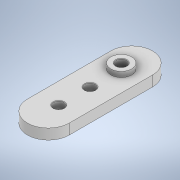
# Autodesk Inventor part: Board
Saved by Autodesk Inventor 2022 (Build 260153000, 153)
## iProperties
Created: 2021-09-18
Part Number: Board
Material: Generic
Document SubType Name: Modeling
Designer: marcu
Density: 1 g/cm^3
Appearance: Default
Author: marcu
Autodesk Inventor part; units mm, degrees
ref_plane "YZ Plane" through (0, 0, 0) normal (1, 0, 0) x (0, 1, 0)
ref_plane "XZ Plane" through (0, 0, 0) normal (0, 1, 0) x (-1, 0, 0)
ref_plane "XY Plane" through (0, 0, 0) normal (0, 0, 1) x (1, 0, 0)
sketch "Sketch1" plane through (0, 0, 0) normal (0, 1, 0) x (-1, 0, 0)
  line L0 (0, 0) -> (25.4, 0)
  line L1 (25.4, 0) -> (25.4, -76.2)
  line L2 (25.4, -76.2) -> (0, -76.2)
  line L3 (0, -76.2) -> (0, 0)
  dimension "d0" = 25.4
  dimension "d1" = 76.2
  constraints: 8 end point, 2 parallel, 1 horizontal, 1 perpendicular
  measures "d0" distance of L1.end L2.end
  measures "d1" distance of L0.end L1.end
extrude "Extrusion1" add sketch "Sketch1" along normal blind 3.175
sketch "Sketch2" plane through (0, 3.175, 0) normal (0, 1, 0) x (1, 0, 0)
  line L0 (-25.4, 76.2) -> (-25.4, 0) projected
  line L1 (0, 76.2) -> (-25.4, 76.2) projected
  line L2 (-25.4, 0) -> (0, 76.2)
  line L3 (0, 76.2) -> (-25.4, 76.2)
  line L4 (-25.4, 76.2) -> (0, 0)
  line L5 (0, 0) -> (-12.7, 38.1)
  line L6 (-25.4, 0) -> (0, 0) projected
  line L7 (-12.7, 0) -> (-12.7, 76.2)
  circle A0 centre (-12.7, 38.1) radius 3.175
  line L8 (-12.7, 38.1) -> (-12.7, 0)
  circle A1 centre (-12.7, 19.05) radius 3.175
  line L9 (-12.7, 38.1) -> (-12.7, 76.2)
  circle A2 centre (-12.7, 57.15) radius 3.175
  dimension "d4" = 6.35
  dimension "d5" = 6.35
  dimension "d6" = 6.35
  constraints: 14 end point, 5 midpoint, 3 centre point, 2 collinear, 1 coincident, 1 horizontal
  measures "d4" diameter of A0
  measures "d5" diameter of A1
  measures "d6" diameter of A2
extrude "Extrusion2" cut sketch "Sketch2" against normal blind 3.175 contours A0 L7 L4 | L4 L2 A0 | L2 L7 A0 | A2 L7 | L7 A2 | L7 A0 L2 | L2 A0 L4 | L4 A0 L7 | A1 L7 | L7 A1
fillet "Fillet1" radius 12.7 4 edges at (0, 1.5875, 0) (-25.4, 1.5875, 0) (0, 1.5875, -76.2) (-25.4, 1.5875, -76.2)
fillet "Fillet2" radius 0.3175 3 edges at (-15.875, 3.175, -57.15) (-15.875, 3.175, -38.1) (-15.875, 3.175, -19.05)
sketch "Sketch3" plane through (0, 3.175, 0) normal (0, 1, 0) x (1, 0, 0)
  circle A0 centre (-12.7, 57.15) radius 3.175 projected
  circle A1 centre (-12.7, 57.15) radius 6.35
  point P0 (0, 0)
  dimension "d11" = 12.7
  constraints: 1 centre point, 1 coincident
  measures "d11" diameter of A1
extrude "Extrusion3" add sketch "Sketch3" along normal blind 3.175
sketch "Sketch4" plane through (-12.7, 6.35, -57.15) normal (0, 1, 0) x (1, 0, 0)
  circle A0 centre (0, 0) radius 6.35 projected
  circle A1 centre (0, 0) radius 3.175 projected
  point P0 (12.7, -57.15)
extrude "Extrusion4" add sketch "Sketch4" against normal through all
fillet "Fillet3" radius 0.3175 1 edges at (-15.875, 6.35, -57.15)
sketch "Sketch5" plane through (0, 0, 0) normal (0, -1, 0) x (1, 0, 0)
  circle A0 centre (-12.7, -38.1) radius 3.175 projected
  circle A1 centre (-12.7, -19.05) radius 3.175 projected
  arc A2 (-25.4, -63.5) -> (0, -63.5) centre (-12.7, -63.5) ccw projected
  line L0 (0, -12.7) -> (0, -63.5) projected
  arc A3 (0, -12.7) -> (-25.4, -12.7) centre (-12.7, -12.7) ccw projected
  line L1 (-25.4, -63.5) -> (-25.4, -12.7) projected
  circle A4 centre (-12.7, -57.15) radius 3.175 projected
  point P0 (0, 0)
extrude "Extrusion5" add sketch "Sketch5" along normal blind 3.175
sketch "Sketch6" plane through (0, -3.175, 0) normal (0, -1, 0) x (1, 0, 0)
  line L0 (-25.4, -12.7) -> (-25.4, -63.5) projected
  arc A0 (-25.4, -63.5) -> (0, -63.5) centre (-12.7, -63.5) ccw projected
  line L1 (0, -63.5) -> (0, -12.7) projected
  arc A1 (0, -12.7) -> (-25.4, -12.7) centre (-12.7, -12.7) ccw projected
  circle A2 centre (-12.7, -57.15) radius 3.175 projected
  circle A3 centre (-12.7, -19.05) radius 3.175 projected
  circle A4 centre (-12.7, -38.1) radius 3.175 projected
  circle A5 centre (-12.7, -57.15) radius 3.175
  circle A6 centre (-12.7, -57.15) radius 3.1877
  circle A7 centre (-12.7, -38.1) radius 3.175
  circle A8 centre (-12.7, -38.1) radius 3.175 projected
  circle A9 centre (-12.7, -38.1) radius 3.1877
  circle A10 centre (-12.7, -19.05) radius 3.175
  circle A11 centre (-12.7, -19.05) radius 3.175
  circle A12 centre (-12.7, -19.05) radius 3.1877
  point P0 (0, 0)
  dimension "d19" = 6.3754
  dimension "d20" = 6.3754
  dimension "d21" = 6.3754
  constraints: 7 centre point, 7 coincident, 1 concentric
  measures "d19" diameter of A6
  measures "d20" diameter of A9
  measures "d21" diameter of A12
extrude "Extrusion6" cut sketch "Sketch6" against normal blind 25.4 contours A2 | A3 | A4 | A6 | A9 | A12
body "Solid1"
